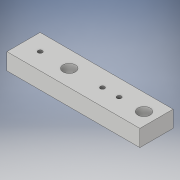
# Autodesk Inventor part: LFEV2017_TSI_004
Saved by Autodesk Inventor 2017 (Build 210142000, 142)
## iProperties
Created: 2017-03-02
Part Number: LFEV2017_TSI_004
Material: Generic
Document SubType Name: Modeling
Designer: coffmant
Density: 1 g/cm^3
Appearance: Default
Author: coffmant
Autodesk Inventor part; units mm, degrees
ref_plane "YZ Plane" through (0, 0, 0) normal (1, 0, 0) x (0, 1, 0)
ref_plane "XZ Plane" through (0, 0, 0) normal (0, 1, 0) x (-1, 0, 0)
ref_plane "XY Plane" through (0, 0, 0) normal (0, 0, 1) x (1, 0, 0)
sketch "Sketch1" plane through (0, 0, 0) normal (1, 0, 0) x (0, 1, 0)
  line L0 (0, 0) -> (12.7, 0)
  line L1 (12.7, 0) -> (12.7, -25.4)
  line L2 (12.7, -25.4) -> (0, -25.4)
  line L3 (0, -25.4) -> (0, 0)
  dimension "d0" = 12.7
  dimension "d1" = 25.4
  constraints: 8 end point, 2 parallel, 1 horizontal, 1 perpendicular
  measures "d0" distance between parallel lines of L3 L1
  measures "d1" distance between parallel lines of L0 L2
extrude "Extrusion1" add sketch "Sketch1" along normal blind 76.2
sketch "Sketch2" plane through (0, 12.7, 0) normal (0, 1, 0) x (1, 0, 0)
  circle A0 centre (9.525, 12.7) radius 4.7625
  line L0 (0, 0) -> (76.2, 0) projected
  line L1 (0, 25.4) -> (76.2, 25.4) projected
  line L2 (0, 0) -> (0, 25.4) projected
  circle A1 centre (66.675, 12.7) radius 4.7625
  line L3 (76.2, 25.4) -> (76.2, 0) projected
  dimension "d4" = 12.7
  dimension "d5" = 25.4
  dimension "d6" = 9.525
  dimension "d7" = 4.7625
  dimension "d8" = 9.525
  dimension "d9" = 12.7
  dimension "d10" = 4.7625
  constraints: 2 centre point
  measures "d4" distance from line of L0 A0.centre
  measures "d5" distance between parallel lines of L1 L0
  measures "d6" diameter of A0
  measures "d7" distance edge to line of A0 L2
  measures "d8" diameter of A1
  measures "d9" distance from line of L0 A1.centre
  measures "d10" distance edge to line of A1 L3
extrude "Extrusion2" cut sketch "Sketch2" against normal through all contours A0 | A1
sketch "Sketch5" plane through (0, 12.7, 0) normal (0, 1, 0) x (1, 0, 0)
  line L0 (0, 0) -> (76.2, 0) projected
  line L1 (0, 25.4) -> (76.2, 25.4) projected
  circle A0 centre (66.675, 12.7) radius 4.7625 projected
  point P0 (47.625, 12.7)
  dimension "d26" = 12.7
  dimension "d27" = 25.4
  dimension "d28" = 19.05
  measures "d26" distance from line of L0 point (47.625, 12.7)
  measures "d27" distance between parallel lines of L0 L1
  measures "d28" distance of A0.centre point (47.625, 12.7)
hole "Hole2" at (47.625, 12.7, -12.7) direction (0, -1, 0) diameter 3.302 end through all thread size "8-32 UNC" class "2B" standard "ANSI Unified Screw Threads"
sketch "Sketch7" plane through (0, 0, 0) normal (-1, 0, 0) x (0, 0, 1)
  line L0 (-25.4, 12.7) -> (-25.4, 0) projected
  line L1 (0, 12.7) -> (-25.4, 12.7) projected
  line L2 (-25.4, 0) -> (0, 0)
  line L3 (0, 0) -> (0, 12.7)
  line L4 (0, 12.7) -> (-25.4, 12.7)
  line L5 (-25.4, 12.7) -> (-25.4, 0)
  point P0 (0, 0)
  constraints: 8 end point, 2 parallel, 1 horizontal, 1 perpendicular
extrude "Extrusion4" add sketch "Sketch7" along normal blind 25.4
sketch "Sketch10" plane through (-25.4, 12.7, -25.4) normal (0, 1, 0) x (1, 0, 0)
  circle A0 centre (73.025, -12.7) radius 1.651 projected
  circle A1 centre (34.925, -12.7) radius 4.7625 projected
  circle A2 centre (92.075, -12.7) radius 4.7625 projected
  line L0 (101.6, 0) -> (101.6, -25.4) projected
  line L1 (101.6, 0) -> (0, 0) projected
  line L2 (0, -25.4) -> (0, 0) projected
  line L3 (101.6, -25.4) -> (0, -25.4) projected
  point P0 (25.4, -25.4)
  point P1 (12.7, -12.7)
  point P2 (88.9, -38.1)
  dimension "d56" = 25.4
  dimension "d58" = 12.7
  dimension "d61" = 12.7
  measures "d56" distance between parallel lines of L1 L3
  measures "d58" distance from line of point (12.7, -12.7) L3
  measures "d61" distance from line of point (12.7, -12.7) L2
hole "Hole4" at (-12.7, 12.7, -12.7) at (63.5, 12.7, 12.7) direction (0, -1, 0) diameter 3.302 end through all thread size "8-32 UNC" class "2B" standard "ANSI Unified Screw Threads"
sketch "Sketch11" plane through (76.2, 12.7, 0) normal (0, 1, 0) x (1, 0, 0)
  circle A0 centre (-88.9, 12.7) radius 1.651 projected
  circle A1 centre (-28.575, 12.7) radius 1.651 projected
  circle A2 centre (-66.675, 12.7) radius 4.7625 projected
  circle A3 centre (-9.525, 12.7) radius 4.7625 projected
  line L0 (0, 0) -> (-101.6, 0) projected
  line L1 (0, 25.4) -> (0, 0) projected
  line L2 (0, 25.4) -> (-101.6, 25.4) projected
  line L3 (-101.6, 0) -> (-101.6, 25.4) projected
  point P0 (-76.2, 0)
  point P1 (-41.275, 12.7)
  dimension "d73" = 12.7
  dimension "d74" = 12.7
  dimension "d75" = 12.7
  measures "d73" distance of point (-41.275, 12.7) A1.centre
  measures "d74" distance from line of A1.centre L0
  measures "d75" distance from line of point (-41.275, 12.7) L0
hole "Hole5" at (34.925, 12.7, -12.7) direction (0, -1, 0) diameter 3.302 end through all thread size "8-32 UNC" class "2B" standard "ANSI Unified Screw Threads"
equation "\"d4\" = 0.5 * d5"
equation "\"d8\" = d6"
equation "\"d9\" = d4"
equation "\"d10\" = d7"
equation "\"d26\" = 0.5 * d27"
equation "\"d58\" = 0.5 * d56"
equation "\"d75\" = d74"
body "Solid1"
